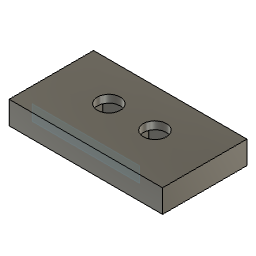
Rail limit sensor holder (Autodesk Fusion 360 archive; units mm, degrees)
design "Testi rail sensorin pidike"
Autodesk Fusion 360 part; units mm, degrees
sketch "Sketch1" plane through (0, 0, 0) normal (0, 0, 1) x (1, 0, 0)
  line L0 (0, 0) -> (14, 0)
  line L1 (14, 0) -> (14, 11)
  line L2 (14, 11) -> (0, 11)
  line L3 (0, 11) -> (0, 0)
  dimension "d1" = 14
  dimension "d2" = 11
  constraint horizontal L0
  constraint vertical L1
  constraint horizontal L2
  constraint vertical L3
  constraint coincident L0.start L3.end
  measures "d1" distance of L0.start L0.end
  measures "d2" distance of L0.start L2.end
extrude "Extrude1" add sketch "Sketch1" along normal blind 2
sketch "Sketch2" plane through (0, 0, 0) normal (0, -1, 0) x (1, 0, 0)
  line L0 (0, 0) -> (14, 0)
  line L1 (14, 0) -> (14, 2)
  line L2 (14, 2) -> (0, 2)
  line L3 (0, 2) -> (0, 0)
sketch "Sketch3" plane through (0, 0, 2) normal (0, 0, 1) x (-1, 0, 0)
  line L0 (0, -11) -> (0, 0)
  line L1 (0, 0) -> (-14, 0)
  line L2 (-14, 0) -> (-14, -11)
  line L3 (-14, -11) -> (0, -11)
  line L4 (0, -11) -> (3, -11)
  line L5 (3, -11) -> (3, 0)
  line L6 (3, 0) -> (0, 0)
  line L7 (0, 0) -> (0, -11)
  line L8 (-14, -11) -> (-17, -11)
  line L9 (-17, -11) -> (-17, 0)
  line L10 (-17, 0) -> (-14, 0)
  line L11 (-14, 0) -> (-14, -11)
  dimension "d26" = 3
  dimension "d27" = 3
  constraint horizontal L4
  constraint vertical L5
  constraint horizontal L6
  constraint vertical L7
  constraint coincident L0.start L3.end
  constraint horizontal L8
  constraint vertical L9
  constraint horizontal L10
  constraint vertical L11
  constraint coincident L2.end L3.start
  measures "d26" distance of L5.end L0.end
  measures "d27" distance of L1.end L9.end
extrude "Extrude2" add sketch "Sketch3" along normal blind 7 and the other way blind 2 contours L0 L4 L5 L6 L7 | L2 L8 L9 L10 L11
sketch "Sketch4" plane through (0, 0, 0) normal (0, 0, -1) x (1, 0, 0)
  line L0 (-3, -11) -> (17, -11)
  line L1 (17, -11) -> (17, 0)
  line L2 (17, 0) -> (-3, 0)
  line L3 (-3, 0) -> (-3, -11)
  line L4 (-3, 0) -> (17, 0)
  line L5 (17, 0) -> (17, -11)
  line L6 (17, -11) -> (-3, -11)
  line L7 (-3, -11) -> (-3, 0)
  constraint horizontal L4
  constraint vertical L5
  constraint horizontal L6
  constraint vertical L7
  constraint coincident L0.end L1.start
  constraint coincident L2.end L3.start
extrude "Extrude3" add sketch "Sketch4" along normal blind 2
sketch "Sketch5" plane through (0, 0, 2) normal (0, 0, 1) x (-1, 0, 0)
  line L0 (0, -11) -> (0, 0)
  line L1 (0, 0) -> (-14, 0)
  line L2 (-14, 0) -> (-14, -11)
  line L3 (-14, -11) -> (0, -11)
  line L4 (-7, -11) -> (-7, -6)
  line L5 (-7, -6) -> (0, -6)
  line L6 (-7, -6) -> (-14, -6)
  circle A0 centre (-4, -6) radius 1.5
  circle A1 centre (-10, -6) radius 1.5
  dimension "d11" = 5
  dimension "d12" = 3
  dimension "d13" = 3
  dimension "d31" = 6
  dimension "d32" = 4
  constraint midpoint L3 L4.start
  constraint perpendicular L3 L4
  constraint coincident L0 L5.end
  constraint perpendicular L0 L5
  constraint coincident L2 L6.end
  constraint perpendicular L2 L6
  constraint coincident L6 A1.centre
  measures "d11" distance of L4.start L4.end
  measures "d12" diameter of A0
  measures "d13" diameter of A1
  measures "d31" distance of A0.centre A1.centre
  measures "d32" distance of L5.end A0.centre
extrude "Extrude4" cut sketch "Sketch5" against normal blind 4 contours L5 A0 | L5 A0 | L6 A1 | L6 A1
sketch "Sketch7" plane through (0, 0, -2) normal (0, 0, -1) x (1, 0, 0)
  circle A0 centre (4, -6) radius 1.5
  circle A1 centre (10, -6) radius 1.5
  line L0 (-3, -11) -> (17, -11)
  line L1 (17, -11) -> (17, 0)
  line L2 (17, 0) -> (-3, 0)
  line L3 (-3, 0) -> (-3, -11)
  line L4 (11.9876, -4.8242) -> (9.9755, -3.6907)
  line L5 (9.9755, -3.6907) -> (7.9879, -4.8666)
  line L6 (7.9879, -4.8666) -> (8.0124, -7.1758)
  line L7 (8.0124, -7.1758) -> (10.0245, -8.3093)
  line L8 (10.0245, -8.3093) -> (12.0121, -7.1334)
  line L9 (12.0121, -7.1334) -> (11.9876, -4.8242)
  line L10 (2.0156, -7.1814) -> (4.0309, -8.3092)
  line L11 (4.0309, -8.3092) -> (6.0153, -7.1278)
  line L12 (6.0153, -7.1278) -> (5.9844, -4.8186)
  line L13 (5.9844, -4.8186) -> (3.9691, -3.6908)
  line L14 (3.9691, -3.6908) -> (1.9847, -4.8722)
  line L15 (1.9847, -4.8722) -> (2.0156, -7.1814)
  point P0 (10, -6)
  point P1 (4, -6)
  dimension "d22" = 2
  dimension "d23" = 2
  constraint coincident P0 A1.centre
  constraint coincident A0.centre P1
  measures "d22" distance of P0 L9
  measures "d23" distance of P1 L15
extrude "Extrude6" cut sketch "Sketch7" against normal blind 2 contours L4 L5 L6 L7 L8 L9 | L10 L11 L12 L13 L14 L15
fillet "Fillet1" radius 1 4 edges at (-3, 5.5, 9) (0, 5.5, 9) (14, 5.5, 9) (17, 5.5, 9)
sketch "Sketch8" plane through (0, 11, 0) normal (0, 1, 0) x (-1, 0, 0)
  arc A0 (-16, 9) -> (-17, 8) centre (-16, 8) ccw
  line L0 (-17, 8) -> (-17, -2)
  line L1 (-17, -2) -> (3, -2)
  line L2 (3, -2) -> (3, 8)
  arc A1 (3, 8) -> (2, 9) centre (2, 8) ccw
  line L3 (2, 9) -> (1, 9)
  arc A2 (1, 9) -> (0, 8) centre (1, 8) ccw
  line L4 (0, 8) -> (0, 2)
  line L5 (0, 2) -> (-14, 2)
  line L6 (-14, 2) -> (-14, 8)
  arc A3 (-14, 8) -> (-15, 9) centre (-15, 8) ccw
  line L7 (-15, 9) -> (-16, 9)
  line L8 (-14, 2) -> (-17, 2)
  line L9 (-17, 2) -> (-17, 9)
  line L10 (-17, 9) -> (-14, 9)
  line L11 (-14, 9) -> (-14, 2)
  line L12 (0, 2) -> (3, 2)
  line L13 (3, 2) -> (3, 9)
  line L14 (3, 9) -> (0, 9)
  line L15 (0, 9) -> (0, 2)
  constraint horizontal L8
  constraint vertical L9
  constraint horizontal L10
  constraint vertical L11
  constraint coincident L5.end L6.start
  constraint horizontal L12
  constraint vertical L13
  constraint horizontal L14
  constraint vertical L15
  constraint coincident L4.end L5.start
extrude "Extrude7" cut sketch "Sketch8" against normal blind 4 contours A0 L0 L6 A3 L7 L8 L9 L10 L11 | L2 A1 L3 A2 L4 L12 L13 L14 L15
fillet "Fillet2" radius 2 1 edges at (7, 11, 2)
delete_face "DeleteFace1" 1 faces at (10.3333, 9.0952, 1.9977)
sketch "Sketch9" plane through (17, 0, 0) normal (1, 0, 0) x (0, 1, 0)
  line L0 (11, 2) -> (7, 2)
  line L1 (7, 2) -> (7, 8)
  line L2 (7, 8) -> (0, 8)
  line L3 (0, 8) -> (0, -2)
  line L4 (0, -2) -> (11, -2)
  line L5 (11, -2) -> (11, 2)
  line L6 (7, 2) -> (0, 2)
  line L7 (0, 2) -> (0, 9)
  line L8 (0, 9) -> (7, 9)
  line L9 (7, 9) -> (7, 2)
  constraint horizontal L6
  constraint vertical L7
  constraint horizontal L8
  constraint vertical L9
  constraint coincident L0.end L1.start
extrude "Extrude8" cut sketch "Sketch9" against normal blind 20 contours L1 L2 L3 L6 L7 L9 | L2 L7 L8 L9
extrude "Extrude9" cut 1 faces at (7.8887, 1.5125, 2) along direction (0, 0, -1) blind 1
